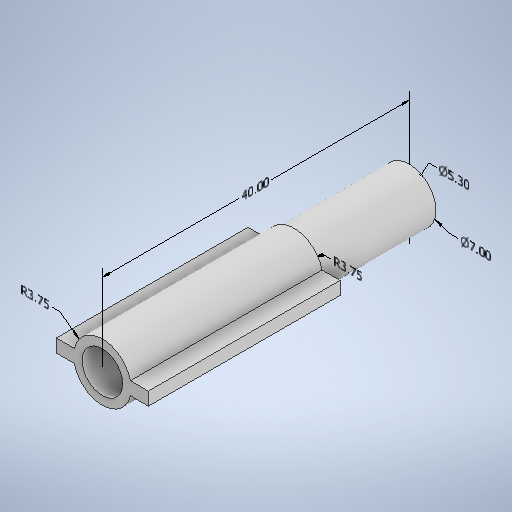
# Autodesk Inventor part: final pin
Saved by Autodesk Inventor 2025.4 (Build 294407000, 407)
## iProperties
Created: 2026-03-10
Part Number: final pin
Material: Generic
Document SubType Name: Modeling
Designer: Amir
Density: 1 g/cm^3
Appearance: Default
Author: Amir
## iProperties of the stored document final pin_3DPrint.ipt
Created: 2026-04-09
Part Number: final pin_3DPrint
Material: Generic
Document SubType Name: Modeling
Designer: Amir
Density: 1 g/cm^3
Appearance: Default
Author: Amir
Autodesk Inventor part; units mm, degrees
ref_plane "YZ Plane" through (0, 0, 0) normal (1, 0, 0) x (0, 1, 0)
ref_plane "XZ Plane" through (0, 0, 0) normal (0, 1, 0) x (-1, 0, 0)
ref_plane "XY Plane" through (0, 0, 0) normal (0, 0, 1) x (1, 0, 0)
sketch "Sketch1" plane through (0, 0, 0) normal (0, 0, 1) x (1, 0, 0)
  circle A0 centre (0, 0) radius 2.65
  circle A1 centre (0, 0) radius 3.5
  dimension "d0" = 5.3
  dimension "d1" = 7
  constraints: 2 centre point, 2 coincident
  measures "d0" diameter of A0
  measures "d1" diameter of A1
extrude "Extrusion1" add sketch "Sketch1" along normal blind 15
sketch "Sketch2" plane through (0, 0, 15) normal (0, 0, 1) x (1, 0, 0)
  circle A0 centre (0, 0) radius 2.65 projected
  circle A1 centre (0, 0) radius 3.75
  line L0 (-6, 0.85) -> (6, 0.85)
  line L1 (6, 0.85) -> (6, -0.85)
  line L2 (6, -0.85) -> (-6, -0.85)
  line L3 (-6, -0.85) -> (-6, 0.85)
  line L4 (-6, 0.85) -> (6, -0.85) construction
  line L5 (6, 0.85) -> (-6, -0.85) construction
  point P0 (-3.6524, 0.85)
  point P1 (-3.6524, -0.85)
  point P2 (3.6524, -0.85)
  point P3 (3.6524, 0.85)
  dimension "d4" = 7.5
  dimension "d5" = 12
  dimension "d6" = 1.7
  constraints: 12 end point, 2 midpoint, 2 parallel, 1 centre point, 1 coincident, 1 horizontal, 1 perpendicular
  measures "d4" diameter of A1
  measures "d5" distance of L1.end L2.end
  measures "d6" distance of L0.end L1.end
extrude "Extrusion2" add sketch "Sketch2" along normal blind 25 contours A0 L0 A1 L2 | A0 L0 A1 | L2 A1 A0 | A0 L2 A1 L0 | L0 L1 L2 A1 | A1 L2 L3 L0
body "Solid1"
